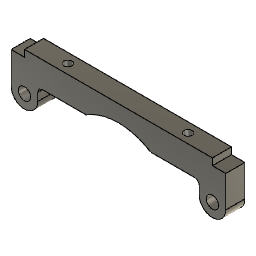
JRCNC0013 v21 (Autodesk Fusion 360 design; units mm, degrees)
Autodesk Fusion 360 part; units mm, degrees
sketch "Sketch1" plane through (0, 0, 0) normal (0, 0, 1) x (1, 0, 0)
  line L0 (71.4, 6.35) -> (-71.4, 6.35)
  line L1 (-71.4, 6.35) -> (-71.4, -6.35)
  line L2 (-71.4, -6.35) -> (71.4, -6.35)
  line L3 (71.4, -6.35) -> (71.4, 6.35)
  line L4 (71.4, 6.35) -> (-71.4, -6.35) construction
  line L5 (-71.4, 6.35) -> (71.4, -6.35) construction
  dimension "d1" = 142.8
  dimension "d2" = 12.7
  constraint horizontal L0
  constraint perpendicular L0 L1
  constraint parallel L0 L2
  constraint parallel L1 L3
  constraint coincident L4 origin
  constraint coincident L5 origin
  measures "d1" distance of L0.start L0.end
  measures "d2" distance of L0.start L2.end
extrude "Extrude1" add sketch "Sketch1" along normal blind 12.7
sketch "Sketch2" plane through (0, 6.35, 0) normal (0, 1, 0) x (-1, 0, 0)
  line L0 (-71.4, 0) -> (71.4, 0)
  line L1 (71.4, 0) -> (71.4, 12.7)
  line L2 (71.4, 12.7) -> (-71.4, 12.7)
  line L3 (-71.4, 12.7) -> (-71.4, 0)
  circle A0 centre (-62.51, -8.3) radius 8.89
  circle A1 centre (62.51, -8.3) radius 8.89
  line L4 (-62.51, -8.3) -> (62.51, -8.3) construction
  line L5 (0, 0) -> (0, -8.3) construction
  line L6 (-71.4, -8.3) -> (-53.62, -8.3)
  line L7 (-53.62, -8.3) -> (-53.62, 12.7)
  line L8 (-53.62, 12.7) -> (-71.4, 12.7)
  line L9 (-71.4, 12.7) -> (-71.4, -8.3)
  line L10 (71.4, -8.3) -> (53.62, -8.3)
  line L11 (53.62, -8.3) -> (53.62, 12.7)
  line L12 (53.62, 12.7) -> (71.4, 12.7)
  line L13 (71.4, 12.7) -> (71.4, -8.3)
  dimension "d6" = 17.78
  dimension "d7" = 17.78
  dimension "d19" = 21
  constraint coincident A0.centre L4.start
  constraint parallel L0 L4
  constraint coincident A1.centre L4.end
  constraint coincident L5.start origin
  constraint perpendicular L0 L5
  constraint midpoint L4 L5.end
  constraint horizontal L6
  constraint vertical L7
  constraint horizontal L8
  constraint vertical L9
  constraint coincident A0 L6.start
  constraint horizontal L10
  constraint vertical L11
  constraint horizontal L12
  constraint vertical L13
  constraint coincident L2 L11.end
  constraint coincident A1 L10.start
  constraint coincident A1 L10.end
  constraint coincident L4 L10.end
  constraint coincident A0 L6.end
  constraint coincident L4 L6.end
  constraint coincident L2.end L3.start
  measures "d6" diameter of A0
  measures "d7" diameter of A1
  measures "d19" distance of A1.centre L12
extrude "Extrude2" add sketch "Sketch2" against normal blind 12.7 contours L0 L2 L3 A0 L7 L8 L9 | L0 A0 L9 | L0 A0 | L0 A0 L6 | A0 L6 | L0 A0 L7 | L0 L1 L2 A1 L11 L12 L13 | L0 A1 L11 | L0 A1 | L0 A1 L10 | A1 L10 | L0 A1 L13
sketch "Sketch3" plane through (0, -6.35, 0) normal (0, -1, 0) x (1, 0, 0)
  line L0 (-53.62, 0) -> (53.62, 0)
  line L1 (53.62, 0) -> (53.62, -8.3)
  arc A0 (53.62, -8.3) -> (71.4, -8.3) centre (62.51, -8.3) ccw
  line L2 (71.4, -8.3) -> (71.4, 12.7)
  line L3 (71.4, 12.7) -> (-71.4, 12.7)
  line L4 (-71.4, 12.7) -> (-71.4, -8.3)
  arc A1 (-71.4, -8.3) -> (-53.62, -8.3) centre (-62.51, -8.3) ccw
  line L5 (-53.62, -8.3) -> (-53.62, 0)
  circle A2 centre (-62.51, -8.3) radius 4.0625
  circle A3 centre (62.51, -8.3) radius 4.0625
  dimension "d11" = 8.125
  dimension "d12" = 8.125
  constraint concentric A1 A2
  constraint concentric A0 A3
  measures "d11" diameter of A3
  measures "d12" diameter of A2
extrude "Extrude3" cut sketch "Sketch3" against normal blind 10 contours A2 | A3
sketch "Sketch4" plane through (0, 0, 0) normal (0, 0, -1) x (1, 0, 0)
  line L0 (-53.62, 6.35) -> (-53.62, -6.35)
  line L1 (-53.62, -6.35) -> (53.62, -6.35)
  line L2 (53.62, -6.35) -> (53.62, 6.35)
  line L3 (53.62, 6.35) -> (-53.62, 6.35)
  line L4 (-40, 0) -> (40, 0)
  dimension "d15" = 80
  constraint parallel L3 L4
  constraint midpoint origin L4
  measures "d15" distance of L4.start L4.end
hole "Hole1" at (-40, 0, 0) at (40, 0, 0) direction (0, 0, 1) diameter 5.5 depth 35 tip angle 180 counterbore diameter 10 counterbore depth 10
fillet "Fillet1" radius 3 2 edges at (-53.62, 0, 0) (53.62, 0, 0)
sketch "Sketch5" plane through (0, 0, 12.7) normal (0, 0, 1) x (-1, 0, 0)
  circle A0 centre (40, 0) radius 2.75
  circle A1 centre (-40, 0) radius 2.75
  line L0 (71.4, 6.35) -> (-71.4, 6.35)
  line L1 (-71.4, 6.35) -> (-71.4, -6.35)
  line L2 (-71.4, -6.35) -> (71.4, -6.35)
  line L3 (71.4, -6.35) -> (71.4, 6.35)
  line L4 (62.5, -6.35) -> (-62.5, -6.35)
  line L5 (-62.5, -6.35) -> (-62.5, 6.35)
  line L6 (-62.5, 6.35) -> (62.5, 6.35)
  line L7 (62.5, 6.35) -> (62.5, -6.35)
  line L8 (62.5, -6.35) -> (-62.5, 6.35) construction
  line L9 (-62.5, -6.35) -> (62.5, 6.35) construction
  dimension "d22" = 125
  constraint horizontal L4
  constraint perpendicular L4 L5
  constraint parallel L4 L6
  constraint parallel L5 L7
  constraint coincident L2 L4.start
  constraint coincident L8 origin
  constraint coincident L9 origin
  measures "d22" distance of L4.start L4.end
extrude "Extrude4" add sketch "Sketch5" along normal blind 4.5 contours L0 L2 L4 L5 L6 L7
sketch "Sketch6" plane through (0, -6.35, 0) normal (0, -1, 0) x (1, 0, 0)
  circle A0 centre (-62.51, -8.3) radius 4.0625
  circle A1 centre (62.51, -8.3) radius 4.0625
  line L0 (-50.62, 0) -> (50.62, 0)
  arc A2 (53.62, -3) -> (50.62, 0) centre (50.62, -3) ccw
  line L1 (53.62, -3) -> (53.62, -8.3)
  arc A3 (53.62, -8.3) -> (71.4, -8.3) centre (62.51, -8.3) ccw
  line L2 (71.4, -8.3) -> (71.4, 12.7)
  line L3 (71.4, 12.7) -> (62.5, 12.7)
  line L4 (62.5, 12.7) -> (62.5, 17.2)
  line L5 (62.5, 17.2) -> (-62.5, 17.2)
  line L6 (-62.5, 17.2) -> (-62.5, 12.7)
  line L7 (-62.5, 12.7) -> (-71.4, 12.7)
  line L8 (-71.4, 12.7) -> (-71.4, -8.3)
  arc A4 (-71.4, -8.3) -> (-53.62, -8.3) centre (-62.51, -8.3) ccw
  line L9 (-53.62, -8.3) -> (-53.62, -3)
  arc A5 (-50.62, 0) -> (-53.62, -3) centre (-50.62, -3) ccw
  line L10 (0, 17.2) -> (0, -33.8)
  circle A6 centre (0, -33.8) radius 40
  dimension "d27" = 51
  dimension "d28" = 80
  constraint midpoint L5 L10.start
  constraint perpendicular L0 L10
  constraint coincident L10.end A6.centre
  measures "d27" distance of L10.start L10.end
  measures "d28" diameter of A6
extrude "Extrude5" cut sketch "Sketch6" against normal blind 24 contours L0 L10 A6 | L0 A6 | L0 L10 A6
